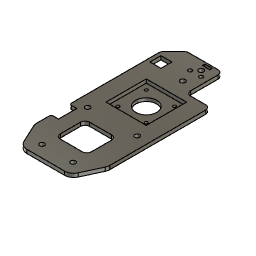
X Axis Support - Motor Side (Autodesk Fusion 360 design; units mm, degrees)
Autodesk Fusion 360 part; units mm, degrees
sketch "Sketch1" plane through (0, 0, 0) normal (0, 0, 1) x (1, 0, 0) in component "X Axis Support - Motor Side"
  line L0 (0, 0) -> (80, 0)
  line L1 (80, 0) -> (80, 180)
  line L2 (80, 180) -> (0, 180)
  line L3 (0, 180) -> (0, 0)
  dimension "d1" = 80
  dimension "d2" = 180
  constraint horizontal L0
  constraint vertical L1
  constraint horizontal L2
  constraint vertical L3
  constraint coincident L0.start L3.end
  measures "d1" distance of L0.start L0.end
  measures "d2" distance of L0.start L2.end
extrude "Extrude1" add sketch "Sketch1" along normal blind 4 in component "X Axis Support - Motor Side"
sketch "Sketch2" plane through (0, 0, 4) normal (0, 0, 1) x (-1, 0, 0) in component "X Axis Support - Motor Side"
  line L0 (0, -180) -> (0, 0)
  line L1 (0, 0) -> (-80, 0)
  line L2 (-80, 0) -> (-80, -180)
  line L3 (-80, -180) -> (0, -180)
  line L4 (-13, -180) -> (-13, 0) construction
  line L5 (-67, -180) -> (-67, 0) construction
  line L6 (-40, -180) -> (-40, 0) construction
  line L7 (0, -13) -> (-80, -13) construction
  line L8 (0, -73) -> (-80, -73) construction
  circle A0 centre (-13, -73) radius 12 construction
  circle A1 centre (-67, -73) radius 12 construction
  circle A2 centre (-13, -73) radius 2.65
  circle A3 centre (-67, -73) radius 2.65
  line L9 (0, -73) -> (0, 0)
  line L10 (0, 0) -> (-40, 0)
  line L11 (-40, 0) -> (-80, 0)
  line L12 (-80, 0) -> (-80, -73)
  line L13 (-23, 0) -> (-23, -180) construction
  line L14 (-57, 0) -> (-57, -180) construction
  circle A4 centre (-23, -13) radius 12 construction
  circle A5 centre (-57, -13) radius 12 construction
  circle A6 centre (-23, -13) radius 2.65
  circle A7 centre (-57, -13) radius 2.65
  line L15 (0, -28) -> (-80, -28) construction
  line L16 (-13, 0) -> (0, -28)
  line L17 (-67, 0) -> (-80, -28)
  line L18 (-23, -28) -> (-57, -28)
  line L19 (-57, -28) -> (-57, -60)
  line L20 (-57, -60) -> (-23, -60)
  line L21 (-23, -60) -> (-23, -28)
  dimension "d5" = 13
  dimension "d6" = 13
  dimension "d7" = 40
  dimension "d8" = 13
  dimension "d13" = 24
  dimension "d14" = 24
  dimension "d16" = 5.3
  dimension "d17" = 5.3
  dimension "d40" = 60
  dimension "d51" = 10
  dimension "d52" = 10
  dimension "d53" = 24
  dimension "d54" = 24
  dimension "d55" = 5.3
  dimension "d56" = 5.3
  dimension "d57" = 28
  dimension "d108" = 34
  dimension "d109" = 32
  constraint coincident L3 L4.start
  constraint coincident L1 L4.end
  constraint perpendicular L1 L4
  constraint coincident L3 L5.start
  constraint coincident L1 L5.end
  constraint perpendicular L1 L5
  constraint coincident L3 L6.start
  constraint coincident L1 L6.end
  constraint perpendicular L1 L6
  constraint coincident L0 L7.start
  constraint coincident L2 L7.end
  constraint perpendicular L2 L7
  constraint coincident L0 L8.start
  constraint coincident L2 L8.end
  constraint perpendicular L2 L8
  constraint coincident L8 A0.centre
  constraint coincident L4 A0.centre
  constraint coincident L8 A1.centre
  constraint coincident L5 A1.centre
  constraint concentric A0 A2
  constraint concentric A1 A3
  constraint coincident L0.end L1.start
  constraint coincident L1.end L2.start
  constraint coincident L10 L13.start
  constraint coincident L3 L13.end
  constraint perpendicular L3 L13
  constraint coincident L11 L14.start
  constraint coincident L3 L14.end
  constraint perpendicular L3 L14
  constraint coincident L13 A4.centre
  constraint coincident L7 A4.centre
  constraint coincident L14 A5.centre
  constraint coincident L7 A5.centre
  constraint concentric A4 A6
  constraint concentric A5 A7
  constraint coincident L9 L15.start
  constraint coincident L12 L15.end
  constraint horizontal L18
  constraint vertical L19
  constraint horizontal L20
  constraint vertical L21
  constraint coincident L15 L18.start
  constraint coincident L13 L18.start
  measures "d5" distance of L0 L4
  measures "d6" distance of L2 L5
  measures "d7" distance of L2 L6
  measures "d8" distance of L1 L7
  measures "d13" diameter of A0
  measures "d14" diameter of A1
  measures "d16" diameter of A2
  measures "d17" diameter of A3
  measures "d40" distance of L7 L8
  measures "d51" distance of L4 L13
  measures "d52" distance of L5 L14
  measures "d53" diameter of A4
  measures "d54" diameter of A5
  measures "d55" diameter of A6
  measures "d56" diameter of A7
  measures "d57" distance of L11 L15
  measures "d108" distance of L18.start L18.end
  measures "d109" distance of L18.start L20.end
extrude "Extrude2" cut sketch "Sketch2" against normal up to surface (4 mm away) contours L0 L1 L9 L10 L16 | L1 L2 L11 L12 L17 | A2 | A3 | A6 | A7 | L18 L19 L20 L21 in component "X Axis Support - Motor Side"
sketch "Sketch14" plane through (0, 0, 4) normal (0, 0, 1) x (-1, 0, 0) in component "X Axis Support - Motor Side"
  line L0 (-67, 0) -> (-80, -28)
  line L1 (-80, -28) -> (-80, -180)
  line L2 (-80, -180) -> (0, -180)
  line L3 (0, -180) -> (0, -28)
  line L4 (0, -28) -> (-13, 0)
  line L5 (-13, 0) -> (-67, 0)
  circle A0 centre (-13, -73) radius 2.65
  circle A1 centre (-57, -13) radius 2.65
  circle A2 centre (-67, -73) radius 2.65
  circle A3 centre (-23, -13) radius 2.65
  line L6 (-23, -60) -> (-57, -60)
  line L7 (-57, -60) -> (-57, -28)
  line L8 (-57, -28) -> (-23, -28)
  line L9 (-23, -28) -> (-23, -60)
  line L10 (0, -66) -> (-80, -66) construction
  line L11 (0, -46) -> (-80, -46) construction
  line L12 (-8, 0) -> (-8, -180) construction
  line L13 (0, -66) -> (-8, -66)
  line L14 (-8, -66) -> (-8, -46)
  line L15 (-8, -46) -> (0, -46)
  line L16 (0, -46) -> (0, -66)
  dimension "d161" = 46
  dimension "d162" = 66
  dimension "d200" = 8
  constraint coincident L3 L10.start
  constraint coincident L1 L10.end
  constraint perpendicular L1 L10
  constraint coincident L3 L11.start
  constraint coincident L1 L11.end
  constraint perpendicular L1 L11
  constraint coincident L5 L12.start
  constraint coincident L2 L12.end
  constraint perpendicular L2 L12
  constraint horizontal L13
  constraint vertical L14
  constraint horizontal L15
  constraint vertical L16
  constraint coincident L11 L14.end
  constraint coincident L12 L14.end
  measures "d161" distance of L5 L11
  measures "d162" distance of L5 L10
  measures "d200" distance of L3 L12
extrude "Extrude13" cut sketch "Sketch14" against normal up to surface (4 mm away) contours L3 L13 L14 L15 L16 in component "X Axis Support - Motor Side"
sketch "Sketch3" plane through (0, 0, 4) normal (0, 0, 1) x (-1, 0, 0) in component "X Axis Support - Motor Side"
  line L0 (-80, -180) -> (0, -180) construction
  line L1 (-40, -180) -> (-40, -30) construction
  line L2 (0, -110) -> (-80, -110) construction
  line L3 (-62, -132) -> (-18, -132)
  line L4 (-18, -132) -> (-18, -88)
  line L5 (-18, -88) -> (-62, -88)
  line L6 (-62, -88) -> (-62, -132)
  line L7 (-62, -132) -> (-18, -88) construction
  line L8 (-18, -132) -> (-62, -88) construction
  line L9 (0, -180) -> (0, -66)
  circle A0 centre (-13, -73) radius 2.65
  circle A1 centre (-67, -73) radius 2.65
  line L10 (-13, -73) -> (-67, -73) construction
  point P0 (-40, -110)
  dimension "d22" = 44
  dimension "d23" = 44
  dimension "d89" = 37
  dimension "d90" = 18
  constraint midpoint L0 L1.start
  constraint perpendicular L0 L1
  constraint horizontal L2
  constraint horizontal L3
  constraint perpendicular L3 L4
  constraint parallel L3 L5
  constraint parallel L4 L6
  constraint coincident L7 P0
  constraint coincident L8 P0
  constraint midpoint L2 P0
  constraint coincident A0.centre L10.start
  constraint coincident A1.centre L10.end
  measures "d22" distance of L4.end L5.end
  measures "d23" distance of L3.end L4.end
  measures "d89" distance of L2 L10
  measures "d90" distance of L4 L9
extrude "Extrude3" cut sketch "Sketch3" against normal up to surface (4 mm away) contours L3 L4 L5 L6 in component "X Axis Support - Motor Side"
fillet "Fillet5" radius 5 4 edges at (23, 60, 2) (57, 60, 2) (57, 28, 2) (23, 28, 2) in component "X Axis Support - Motor Side"
fillet "Fillet5" radius 10 4 edges at (0, 28, 2) (13, 0, 2) (67, 0, 2) (80, 28, 2) in component "X Axis Support - Motor Side"
fillet "Fillet5" radius 2 2 edges at (0, 46, 2) (0, 66, 2) in component "X Axis Support - Motor Side"
sketch "Sketch4" plane through (0, 0, 0) normal (0, 0, -1) x (1, 0, 0) in component "X Axis Support - Motor Side"
  line L0 (18, -88) -> (62, -88)
  line L1 (62, -88) -> (62, -132)
  line L2 (62, -132) -> (18, -132)
  line L3 (18, -132) -> (18, -88)
  circle A0 centre (13, -73) radius 2.65
  circle A1 centre (67, -73) radius 2.65
  line L4 (0, -68) -> (0, -180)
  line L5 (0, -180) -> (80, -180)
  line L6 (15, -135) -> (15, -85)
  line L7 (15, -85) -> (65, -85)
  line L8 (65, -85) -> (65, -135)
  line L9 (65, -135) -> (15, -135)
  line L10 (60.6176, 0) -> (19.3824, 0)
  line L11 (79.0701, -25.9971) -> (69.6877, -5.7889)
  line L12 (10.3123, -5.7889) -> (0.9299, -25.9971)
  circle A2 centre (23, -13) radius 2.65
  circle A3 centre (57, -13) radius 2.65
  line L13 (52, -60) -> (28, -60)
  line L14 (23, -55) -> (23, -33)
  line L15 (28, -28) -> (52, -28)
  line L16 (57, -33) -> (57, -55)
  arc A4 (23, -55) -> (28, -60) centre (28, -55) ccw
  arc A5 (28, -28) -> (23, -33) centre (28, -33) ccw
  arc A6 (57, -33) -> (52, -28) centre (52, -33) ccw
  arc A7 (52, -60) -> (57, -55) centre (52, -55) ccw
  arc A8 (80, -30.2082) -> (79.0701, -25.9971) centre (70, -30.2082) ccw
  arc A9 (69.6877, -5.7889) -> (60.6176, 0) centre (60.6176, -10) ccw
  arc A10 (19.3824, 0) -> (10.3123, -5.7889) centre (19.3824, -10) ccw
  arc A11 (0.9299, -25.9971) -> (0, -30.2082) centre (10, -30.2082) ccw
  line L17 (80, -180) -> (80, -30.2082)
  line L18 (2, -46) -> (8, -46)
  line L19 (8, -46) -> (8, -66)
  line L20 (8, -66) -> (2, -66)
  arc A12 (2, -66) -> (0, -68) centre (2, -68) ccw
  line L21 (0, -30.2082) -> (0, -44)
  arc A13 (0, -44) -> (2, -46) centre (2, -44) ccw
  dimension "d26" = -3
extrude "Extrude4" add sketch "Sketch4" along normal blind 3.5 contours L0 L1 L2 L3 | L6 L7 L8 L9 in component "X Axis Support - Motor Side"
sketch "Sketch6" plane through (0, 0, -3.5) normal (0, 0, -1) x (1, 0, 0) in component "X Axis Support - Motor Side"
  line L0 (65, -135) -> (65, -85)
  line L1 (65, -85) -> (15, -85)
  line L2 (15, -85) -> (15, -135)
  line L3 (15, -135) -> (65, -135)
  line L4 (40, -135) -> (40, -85) construction
  line L5 (65, -110) -> (15, -110) construction
  circle A0 centre (40, -110) radius 11.5
  line L6 (18, -88) -> (18, -132)
  line L7 (18, -132) -> (62, -132)
  line L8 (62, -88) -> (18, -88)
  line L9 (62, -132) -> (62, -88)
  line L10 (55.5, -125.5) -> (24.5, -125.5) construction
  line L11 (24.5, -125.5) -> (24.5, -94.5) construction
  line L12 (24.5, -94.5) -> (55.5, -94.5) construction
  line L13 (55.5, -94.5) -> (55.5, -125.5) construction
  line L14 (55.5, -125.5) -> (24.5, -94.5) construction
  line L15 (24.5, -125.5) -> (55.5, -94.5) construction
  circle A1 centre (55.5, -125.5) radius 1.65
  circle A2 centre (24.5, -125.5) radius 1.65
  circle A3 centre (55.5, -94.5) radius 1.65
  circle A4 centre (24.5, -94.5) radius 1.65
  point P0 (40, -110)
  dimension "d29" = 23
  dimension "d30" = 31
  dimension "d31" = 31
  dimension "d32" = 3.3
  dimension "d33" = 3.3
  dimension "d34" = 3.3
  dimension "d35" = 3.3
  constraint midpoint L3 L4.start
  constraint midpoint L1 L4.end
  constraint midpoint L0 L5.start
  constraint midpoint L2 L5.end
  constraint midpoint L4 P0
  constraint horizontal L10
  constraint perpendicular L10 L11
  constraint parallel L10 L12
  constraint parallel L11 L13
  constraint coincident L14 P0
  constraint coincident L15 P0
  constraint coincident P0 A0.centre
  constraint coincident L10.start L13.end
  constraint coincident L10.end L11.start
  constraint coincident L12.end L13.start
  constraint coincident L11.end L12.start
  measures "d29" diameter of A0
  measures "d30" distance of L11.end L12.end
  measures "d31" distance of L10.end L11.end
  measures "d32" diameter of A1
  measures "d33" diameter of A2
  measures "d34" diameter of A3
  measures "d35" diameter of A4
extrude "Extrude5" cut sketch "Sketch6" against normal up to surface (3.5 mm away) contours A0 | A1 | A2 | A3 | A4 in component "X Axis Support - Motor Side"
fillet "Fillet3" radius 3 4 edges at (15, 135, -1.75) (15, 85, -1.75) (65, 85, -1.75) (65, 135, -1.75) in component "X Axis Support - Motor Side"
fillet "Fillet4" radius 1.5 tangency weight 1.56093 8 edges at (15.8787, 85.8787, 0) (40, 85, 0) (64.1213, 85.8787, 0) (65, 110, 0) (64.1213, 134.1213, 0) (40, 135, 0) (15.8787, 134.1213, 0) (15, 110, 0) in component "X Axis Support - Motor Side"
sketch "Sketch7" plane through (0, 0, 4) normal (0, 0, 1) x (-1, 0, 0) in component "X Axis Support - Motor Side"
  line L0 (0, -44) -> (0, -30.2082)
  line L1 (-0.9299, -25.9971) -> (-10.3123, -5.7889)
  line L2 (-19.3824, 0) -> (-60.6176, 0)
  line L3 (-69.6877, -5.7889) -> (-79.0701, -25.9971)
  line L4 (-80, -30.2082) -> (-80, -180)
  line L5 (-80, -180) -> (0, -180)
  circle A0 centre (-23, -13) radius 2.65
  circle A1 centre (-67, -73) radius 2.65
  circle A2 centre (-57, -13) radius 2.65
  circle A3 centre (-13, -73) radius 2.65
  line L6 (-62, -88) -> (-18, -88)
  line L7 (-18, -88) -> (-18, -132)
  line L8 (-18, -132) -> (-62, -132)
  line L9 (-62, -132) -> (-62, -88)
  line L10 (-40, -180) -> (-40, 0) construction
  line L11 (-40, -180) -> (-40, 0) construction
  line L12 (0, -160) -> (-80, -160) construction
  line L13 (-50, -180) -> (-30, -180) construction
  line L14 (-30, -180) -> (-30, -140) construction
  line L15 (-30, -140) -> (-50, -140) construction
  line L16 (-50, -140) -> (-50, -180) construction
  line L17 (-50, -180) -> (-30, -140) construction
  line L18 (-30, -180) -> (-50, -140) construction
  line L19 (0, -170) -> (-80, -170) construction
  line L20 (0, -150) -> (-80, -150) construction
  circle A4 centre (-40, -170) radius 2.75
  circle A5 centre (-40, -150) radius 2.75
  line L21 (0, -140) -> (-80, -140) construction
  line L22 (-10, -180) -> (-10, 0) construction
  line L23 (-53.5, -180) -> (-53.5, -140) construction
  line L24 (-53.5, -180) -> (-53.5, -140)
  line L25 (-80, -140) -> (-53.5, -140)
  line L26 (-28, -60) -> (-52, -60)
  line L27 (-57, -55) -> (-57, -33)
  line L28 (-52, -28) -> (-28, -28)
  line L29 (-23, -33) -> (-23, -55)
  arc A6 (-57, -55) -> (-52, -60) centre (-52, -55) ccw
  arc A7 (-52, -28) -> (-57, -33) centre (-52, -33) ccw
  arc A8 (-23, -33) -> (-28, -28) centre (-28, -33) ccw
  arc A9 (-28, -60) -> (-23, -55) centre (-28, -55) ccw
  arc A10 (-79.0701, -25.9971) -> (-80, -30.2082) centre (-70, -30.2082) ccw
  arc A11 (0, -30.2082) -> (-0.9299, -25.9971) centre (-10, -30.2082) ccw
  arc A12 (-10.3123, -5.7889) -> (-19.3824, 0) centre (-19.3824, -10) ccw
  arc A13 (-60.6176, 0) -> (-69.6877, -5.7889) centre (-60.6176, -10) ccw
  line L30 (-10, -150) -> (-4, -150)
  line L31 (-10, -150) -> (-16, -150)
  line L32 (-4, -150) -> (-4, -162)
  line L33 (-16, -150) -> (-16, -162)
  line L34 (-16, -162) -> (-4, -162)
  line L35 (0, -178) -> (-80, -178) construction
  line L36 (-40, -178) -> (-44, -178)
  line L37 (-40, -178) -> (-36, -178)
  line L38 (-36, -178) -> (-36, -175.4)
  line L39 (-44, -178) -> (-44, -175.4)
  line L40 (-36, -175.4) -> (-44, -175.4)
  line L41 (-2, -66) -> (-8, -66)
  line L42 (-8, -66) -> (-8, -46)
  line L43 (-8, -46) -> (-2, -46)
  arc A14 (0, -68) -> (-2, -66) centre (-2, -68) ccw
  arc A15 (-2, -46) -> (0, -44) centre (-2, -44) ccw
  line L44 (0, -180) -> (0, -68)
  point P0 (-40, -160)
  point P1 (-10, -150)
  dimension "d79" = 160
  dimension "d80" = 20
  dimension "d81" = 40
  dimension "d82" = 10
  dimension "d83" = 10
  dimension "d84" = 5.5
  dimension "d85" = 5.5
  dimension "d91" = 40
  dimension "d94" = 180
  dimension "d103" = 3.5
  dimension "d114" = 6
  dimension "d115" = 6
  dimension "d116" = 12
  dimension "d117" = 12
  dimension "d155" = 2
  dimension "d156" = 4
  dimension "d157" = 4
  dimension "d158" = 2.6
  dimension "d159" = 2.6
  dimension "d176" = 30
  constraint midpoint L5 L10.start
  constraint midpoint L2 L10.end
  constraint coincident L5 L10.start
  constraint coincident L2 L10.end
  constraint perpendicular L2 L11
  constraint coincident L0 L12.start
  constraint coincident L4 L12.end
  constraint perpendicular L4 L12
  constraint horizontal L13
  constraint perpendicular L13 L14
  constraint parallel L13 L15
  constraint parallel L14 L16
  constraint coincident L17 P0
  constraint coincident L18 P0
  constraint coincident L11 P0
  constraint coincident L12 P0
  constraint coincident L0 L19.start
  constraint coincident L4 L19.end
  constraint perpendicular L4 L19
  constraint coincident L0 L20.start
  constraint coincident L4 L20.end
  constraint perpendicular L4 L20
  constraint coincident L11 A4.centre
  constraint coincident L19 A4.centre
  constraint coincident L20 A5.centre
  constraint coincident L11 A5.centre
  constraint coincident L0 L21.start
  constraint coincident L4 L21.end
  constraint perpendicular L4 L21
  constraint vertical L22
  constraint coincident L5 L22.start
  constraint coincident L22 P1
  constraint coincident L20 P1
  constraint coincident L5 L23.start
  constraint coincident L21 L23.end
  constraint perpendicular L21 L23
  constraint coincident P1 L30.start
  constraint perpendicular L22 L30
  constraint perpendicular L22 L31
  constraint perpendicular L20 L32
  constraint perpendicular L12 L33
  constraint coincident L0 L35.start
  constraint coincident L4 L35.end
  constraint perpendicular L4 L35
  constraint coincident L35 L36.start
  constraint coincident L11 L36.start
  constraint perpendicular L11 L36
  constraint perpendicular L11 L37
  constraint perpendicular L35 L38
  constraint perpendicular L36 L39
  constraint collinear L10 L11
  measures "d79" distance of L2 L12
  measures "d80" distance of L14.end L15.end
  measures "d81" distance of L13.end L14.end
  measures "d82" distance of L12 L19
  measures "d83" distance of L12 L20
  measures "d84" diameter of A4
  measures "d85" diameter of A5
  measures "d91" distance of L5 L21
  measures "d94" distance of L22.start L22.end
  measures "d103" distance of L16 L23
  measures "d114" distance of P1 L30.end
  measures "d115" distance of P1 L31.end
  measures "d116" distance of L30.end L32.end
  measures "d117" distance of L31.end L33.end
  measures "d155" distance of L5 L35
  measures "d156" distance of L36.start L36.end
  measures "d157" distance of L36.start L37.end
  measures "d158" distance of L37.end L38.end
  measures "d159" distance of L36.end L39.end
  measures "d176" distance of L11 L22
extrude "Extrude7" cut sketch "Sketch7" against normal up to surface (4 mm away) contours L4 L5 L24 L25 | A4 | A5 | L30 L31 L32 L33 L34 | L36 L37 L38 L39 L40 in component "X Axis Support - Motor Side"
fillet "Fillet7" radius 5 3 edges at (53.5, 180, 2) (53.5, 140, 2) (80, 140, 2) in component "X Axis Support - Motor Side"
sketch "Sketch9" plane through (0, 0, 0) normal (0, 0, -1) x (1, 0, 0) in component "X Axis Support - Motor Side"
  spline S0 degree 3 poles (18, -83.5) (17.2716, -83.5) (16.5445, -83.6801) (15.5023, -84.2298) (15.1362, -84.4998) (14.818, -84.818) (14.4998, -85.1362) (14.2298, -85.5023) (13.68, -86.5445) (13.5, -87.2716) (13.5, -88) knots 0 0 0 0 0.218287 0.218287 0.353177 0.353177 0.353177 0.488067 0.488067 0.706355 0.706355 0.706355 0.706355
  line L0 (62, -83.5) -> (18, -83.5)
  spline S1 degree 3 poles (66.5, -88) (66.5, -87.55) (66.4321, -87.1005) (66.0865, -85.9829) (65.7062, -85.3481) (64.611, -84.2403) (63.8526, -83.8142) (62.6973, -83.5407) (62.3489, -83.5) (62, -83.5) knots 15.319061 15.319061 15.319061 15.319061 15.45391 15.45391 15.669669 15.669669 15.920855 15.920855 16.025416 16.025416 16.025416 16.025416
  line L1 (66.5, -132) -> (66.5, -88)
  spline S2 degree 3 poles (62, -136.5) (62.45, -136.5) (62.8995, -136.4321) (64.0171, -136.0865) (64.6519, -135.7062) (65.7597, -134.611) (66.1858, -133.8526) (66.4593, -132.6973) (66.5, -132.3489) (66.5, -132) knots 10.212707 10.212707 10.212707 10.212707 10.347556 10.347556 10.563315 10.563315 10.814501 10.814501 10.919062 10.919062 10.919062 10.919062
  line L2 (18, -136.5) -> (62, -136.5)
  spline S3 degree 3 poles (13.5, -132) (13.5, -132.45) (13.5679, -132.8995) (13.9135, -134.0171) (14.2938, -134.6519) (15.389, -135.7597) (16.1474, -136.1858) (17.3027, -136.4593) (17.6511, -136.5) (18, -136.5) knots 5.106353 5.106353 5.106353 5.106353 5.241202 5.241202 5.456961 5.456961 5.708147 5.708147 5.812708 5.812708 5.812708 5.812708
  line L3 (13.5, -88) -> (13.5, -132)
  line L4 (52, -60) -> (28, -60)
  arc A0 (23, -55) -> (28, -60) centre (28, -55) ccw
  line L5 (23, -55) -> (23, -33)
  arc A1 (28, -28) -> (23, -33) centre (28, -33) ccw
  line L6 (28, -28) -> (52, -28)
  arc A2 (57, -33) -> (52, -28) centre (52, -33) ccw
  line L7 (57, -33) -> (57, -55)
  arc A3 (52, -60) -> (57, -55) centre (52, -55) ccw
  circle A4 centre (23, -13) radius 2.65
  circle A5 centre (67, -73) radius 2.65
  circle A6 centre (57, -13) radius 2.65
  circle A7 centre (13, -73) radius 2.65
  line L8 (4, -162) -> (4, -150)
  line L9 (4, -150) -> (16, -150)
  line L10 (16, -150) -> (16, -162)
  line L11 (16, -162) -> (4, -162)
  circle A8 centre (40, -150) radius 2.75
  circle A9 centre (40, -170) radius 2.75
  line L12 (0, -180) -> (48.5, -180)
  arc A10 (48.5, -180) -> (53.5, -175) centre (48.5, -175) ccw
  line L13 (53.5, -175) -> (53.5, -145)
  arc A11 (58.5, -140) -> (53.5, -145) centre (58.5, -145) ccw
  line L14 (58.5, -140) -> (75, -140)
  arc A12 (75, -140) -> (80, -135) centre (75, -135) ccw
  line L15 (80, -135) -> (80, -30.2082)
  arc A13 (80, -30.2082) -> (79.0701, -25.9971) centre (70, -30.2082) ccw
  line L16 (79.0701, -25.9971) -> (69.6877, -5.7889)
  arc A14 (69.6877, -5.7889) -> (60.6176, 0) centre (60.6176, -10) ccw
  line L17 (60.6176, 0) -> (19.3824, 0)
  arc A15 (19.3824, 0) -> (10.3123, -5.7889) centre (19.3824, -10) ccw
  line L18 (10.3123, -5.7889) -> (0.9299, -25.9971)
  arc A16 (0.9299, -25.9971) -> (0, -30.2082) centre (10, -30.2082) ccw
  line L19 (0, -30.2082) -> (0, -44)
  line L20 (44, -175.4) -> (44, -178)
  line L21 (44, -178) -> (36, -178)
  line L22 (36, -178) -> (36, -175.4)
  line L23 (36, -175.4) -> (44, -175.4)
  line L24 (16, -162) -> (4, -162)
  line L25 (4, -150) -> (16, -150)
  line L26 (16, -150) -> (16, -162)
  line L27 (4, -162) -> (4, -150)
  line L28 (10, -162) -> (10, -150) construction
  line L29 (10, -150) -> (20, -150)
  line L30 (10, -150) -> (0, -150)
  line L31 (20, -150) -> (20, -146)
  line L32 (20, -146) -> (0, -146)
  line L33 (0, -150) -> (0, -146)
  line L34 (2, -46) -> (8, -46)
  line L35 (8, -46) -> (8, -66)
  line L36 (8, -66) -> (2, -66)
  line L37 (0, -68) -> (0, -180)
  arc A17 (0, -44) -> (2, -46) centre (2, -44) ccw
  arc A18 (2, -66) -> (0, -68) centre (2, -68) ccw
  dimension "d171" = 10
  dimension "d172" = 10
  dimension "d173" = 4
  dimension "d174" = 20
  constraint midpoint L24 L28.start
  constraint midpoint L25 L28.end
  constraint perpendicular L28 L29
  constraint perpendicular L28 L30
  constraint perpendicular L29 L31
  constraint perpendicular L19 L32
  measures "d171" distance of L28.end L29.end
  measures "d172" distance of L28.end L30.end
  measures "d173" distance of L29.end L31.end
  measures "d174" distance of L31.end L32.end
extrude "Extrude8" add sketch "Sketch9" along normal blind 25 contours L9 L25 L29 L30 L31 L32 L33 L37 in component "X Axis Support - Motor Side"
sketch "Sketch10" plane through (0, 0, 0) normal (-1, 0, 0) x (0, -1, 0) in component "X Axis Support - Motor Side"
  line L0 (-146, 0) -> (-150, 0)
  line L1 (-150, 0) -> (-150, -20)
  line L2 (-150, -20) -> (-146, -20)
  line L3 (-146, -20) -> (-146, 0)
  line L4 (-146, 0) -> (-146, -20)
  line L5 (-146, 0) -> (-139.4987, 0)
  line L6 (-139.4987, 0) -> (-146, -20)
  line L7 (-180, 0) -> (-150, 0)
  line L8 (-150, 0) -> (-150, -25)
  line L9 (-150, -25) -> (-146, -25)
  line L10 (-146, -25) -> (-146, 0)
  line L11 (-146, 0) -> (-68, 0)
  line L12 (-68, 4) -> (-180, 4)
  line L13 (-180, 4) -> (-180, 0)
  line L14 (-68, 0) -> (-68, 4)
  constraint coincident L0.start L3.end
  constraint coincident L2.end L3.start
  constraint perpendicular L4 L5
extrude "Extrude9" add sketch "Sketch10" against normal blind 1.5 contours L3 L4 L5 L6 L10 L11 in component "X Axis Support - Motor Side"
sketch "Sketch11" plane through (20, 0, 0) normal (1, 0, 0) x (0, 1, 0) in component "X Axis Support - Motor Side"
  line L0 (150, 0) -> (146, 0)
  line L1 (146, 0) -> (146, -20)
  line L2 (146, -20) -> (150, -20)
  line L3 (150, -20) -> (150, 0)
  line L4 (146, 0) -> (139.4987, 0)
  line L5 (139.4987, 0) -> (146, -20)
  line L6 (146, 0) -> (146, -20)
  line L7 (150, 0) -> (146, 0)
  line L8 (146, 0) -> (146, -25)
  line L9 (146, -25) -> (150, -25)
  line L10 (150, -25) -> (150, 0)
  constraint coincident L0.end L1.start
  constraint perpendicular L1 L4
  constraint coincident L1.end L2.start
extrude "Extrude10" add sketch "Sketch11" against normal blind 1.5 contours L1 L4 L5 L6 L8 in component "X Axis Support - Motor Side"
fillet "Fillet8" radius 0.75 5 edges at (10, 146, 0) (18.5, 142.7493, 0) (19.25, 139.4987, 0) (0.75, 139.4987, 0) (1.5, 142.7493, 0) in component "X Axis Support - Motor Side"
sketch "Sketch12" plane through (0, 146, 0) normal (0, 1, 0) x (-1, 0, 0) in component "X Axis Support - Motor Side"
  line L0 (-4, 0) -> (-4, 4)
  line L1 (-4, 4) -> (-16, 4)
  line L2 (-16, 4) -> (-16, 0)
  line L3 (-10, -24) -> (-10, -4) construction
  line L4 (-16, 0) -> (-4, 0) construction
  line L5 (-10, -14) -> (-16, -14) construction
  line L6 (-16, -9) -> (-4, -9) construction
  line L7 (-16, -19) -> (-4, -19) construction
  circle A0 centre (-10, -9) radius 2.05
  circle A1 centre (-10, -19) radius 2.05
  line L8 (-16, 0) -> (-20, 0)
  line L9 (-20, 0) -> (-20, -24)
  line L10 (-20, -24) -> (0, -24)
  line L11 (0, -24) -> (0, 0)
  line L12 (0, 0) -> (-4, 0)
  line L13 (-18.5, -0.75) -> (-1.5, -0.75)
  line L14 (-1.5, -0.75) -> (-1.5, -20)
  line L15 (-1.5, -20) -> (0, -20)
  line L16 (0, -20) -> (0, -25)
  line L17 (0, -25) -> (-20, -25)
  line L18 (-20, -25) -> (-20, -20)
  line L19 (-20, -20) -> (-18.5, -20)
  line L20 (-18.5, -20) -> (-18.5, -0.75)
  dimension "d129" = 5
  dimension "d130" = 5
  dimension "d131" = 4.1
  dimension "d132" = 4.1
  dimension "d175" = 9
  constraint coincident L2.end L4.start
  constraint coincident L0.start L4.end
  constraint midpoint L3 L5.start
  constraint midpoint L6 A0.centre
  constraint midpoint L7 A1.centre
  measures "d129" distance of L5 L7
  measures "d130" distance of L5 L6
  measures "d131" diameter of A0
  measures "d132" diameter of A1
  measures "d175" distance of L6 L8
extrude "Extrude11" cut sketch "Sketch12" along normal up to surface (4 mm away) contours A0 | A1 in component "X Axis Support - Motor Side"
sketch "Sketch15" plane through (0, 0, 4) normal (0, 0, 1) x (-1, 0, 0) in component "X Axis Support - Motor Side"
  line L0 (-28, -60) -> (-52, -60)
  arc A0 (-57, -55) -> (-52, -60) centre (-52, -55) ccw
  line L1 (-57, -55) -> (-57, -33)
  arc A1 (-52, -28) -> (-57, -33) centre (-52, -33) ccw
  line L2 (-52, -28) -> (-28, -28)
  arc A2 (-23, -33) -> (-28, -28) centre (-28, -33) ccw
  line L3 (-23, -33) -> (-23, -55)
  arc A3 (-28, -60) -> (-23, -55) centre (-28, -55) ccw
  circle A4 centre (-23, -13) radius 2.65
  circle A5 centre (-67, -73) radius 2.65
  circle A6 centre (-57, -13) radius 2.65
  circle A7 centre (-13, -73) radius 2.65
  line L4 (-62, -88) -> (-18, -88)
  line L5 (-18, -88) -> (-18, -132)
  line L6 (-18, -132) -> (-62, -132)
  line L7 (-62, -132) -> (-62, -88)
  line L8 (-44, -178) -> (-44, -175.4)
  line L9 (-44, -175.4) -> (-36, -175.4)
  line L10 (-36, -175.4) -> (-36, -178)
  line L11 (-36, -178) -> (-44, -178)
  circle A8 centre (-40, -150) radius 2.75
  line L12 (-4, -150) -> (-4, -162)
  line L13 (-4, -162) -> (-16, -162)
  line L14 (-16, -162) -> (-16, -150)
  line L15 (-16, -150) -> (-4, -150)
  circle A9 centre (-40, -170) radius 2.75
  line L16 (0, -180) -> (0, -68)
  arc A10 (0, -30.2082) -> (-0.9299, -25.9971) centre (-10, -30.2082) ccw
  line L17 (-0.9299, -25.9971) -> (-10.3123, -5.7889)
  arc A11 (-10.3123, -5.7889) -> (-19.3824, 0) centre (-19.3824, -10) ccw
  line L18 (-19.3824, 0) -> (-60.6176, 0)
  arc A12 (-60.6176, 0) -> (-69.6877, -5.7889) centre (-60.6176, -10) ccw
  line L19 (-69.6877, -5.7889) -> (-79.0701, -25.9971)
  arc A13 (-79.0701, -25.9971) -> (-80, -30.2082) centre (-70, -30.2082) ccw
  line L20 (-80, -30.2082) -> (-80, -135)
  arc A14 (-80, -135) -> (-75, -140) centre (-75, -135) ccw
  line L21 (-75, -140) -> (-58.5, -140)
  arc A15 (-53.5, -145) -> (-58.5, -140) centre (-58.5, -145) ccw
  line L22 (-53.5, -145) -> (-53.5, -175)
  arc A16 (-53.5, -175) -> (-48.5, -180) centre (-48.5, -175) ccw
  line L23 (-48.5, -180) -> (0, -180)
  line L24 (-40, -170) -> (-40, -150) construction
  line L25 (-40, -164) -> (-53.5, -164) construction
  line L26 (-40, -164) -> (0, -164) construction
  line L27 (-46, -164) -> (-46, -180) construction
  line L28 (-34, -164) -> (-34, -180) construction
  circle A17 centre (-46, -164) radius 2.05
  circle A18 centre (-34, -164) radius 2.05
  line L29 (-53.5, -157) -> (-28.5, -157) construction
  line L30 (-53.5, -161) -> (-28.5, -161) construction
  line L31 (-28.5, -161) -> (-28.5, -167) construction
  line L32 (-28.5, -167) -> (-30.5, -167) construction
  line L33 (-30.5, -167) -> (-30.5, -161) construction
  line L34 (-28.5, -157) -> (-28.5, -161) construction
  line L35 (-2, -66) -> (-8, -66)
  line L36 (-8, -66) -> (-8, -46)
  line L37 (-8, -46) -> (-2, -46)
  arc A19 (0, -68) -> (-2, -66) centre (-2, -68) ccw
  arc A20 (-2, -46) -> (0, -44) centre (-2, -44) ccw
  line L38 (0, -44) -> (0, -30.2082)
  dimension "d179" = 4.1
  dimension "d180" = 4.1
  dimension "d181" = 16
  dimension "d183" = 25
  dimension "d184" = 25
  dimension "d185" = 4
  dimension "d187" = 6
  dimension "d188" = 2
  dimension "d192" = 6
  dimension "d193" = 6
  dimension "d194" = 23
  constraint coincident A9.centre L24.start
  constraint coincident A8.centre L24.end
  constraint perpendicular L16 L26
  constraint coincident L25 L27.start
  constraint coincident L23 L27.end
  constraint perpendicular L23 L27
  constraint coincident L26 L28.start
  constraint coincident L23 L28.end
  constraint perpendicular L23 L28
  constraint coincident L27.start A17.centre
  constraint coincident L28.start A18.centre
  constraint perpendicular L22 L29
  constraint coincident L22 L30.start
  constraint perpendicular L28 L30
  constraint perpendicular L30 L31
  constraint perpendicular L31 L32
  constraint coincident L30 L33.end
  constraint perpendicular L30 L33
  constraint perpendicular L30 L34
  measures "d179" diameter of A17
  measures "d180" diameter of A18
  measures "d181" distance of L23 L25
  measures "d183" distance of L29.start L29.end
  measures "d184" distance of L30.start L30.end
  measures "d185" distance of L29 L30
  measures "d187" distance of L30.end L31.end
  measures "d188" distance of L31.end L32.end
  measures "d192" distance of L24 L28
  measures "d193" distance of L24 L27
  measures "d194" distance of L23 L29
extrude "Extrude14" cut sketch "Sketch15" against normal up to surface (4 mm away) contours A17 | A18 in component "X Axis Support - Motor Side"
chamfer "Chamfer1" distance 14 angle 45 1 edges at (0, 180, 2) in component "X Axis Support - Motor Side"
fillet "Fillet9" radius 5 2 edges at (14, 180, 2) (0, 166, 2) in component "X Axis Support - Motor Side"
component "X Axis Support - Motor Side" placed x (1, 0, 0) y (0, 1, 0) z (0, 0, 1) at (0, 0, 0)
named bodies: "X Axis Support - Motor Side"
